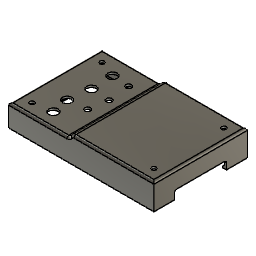
top command (Autodesk Fusion 360 design; units mm, degrees)
Autodesk Fusion 360 part; units mm, degrees
sketch "Esquisse1" plane through (0, 0, 0) normal (0, 0, 1) x (1, 0, 0)
  line L0 (-14.2692, 23.2767) -> (125.7308, 23.2767)
  line L1 (125.7308, 23.2767) -> (125.7308, -66.7233)
  line L2 (125.7308, -66.7233) -> (-14.2692, -66.7233)
  line L3 (-14.2692, -66.7233) -> (-14.2692, 23.2767)
  dimension "d1" = 140
  dimension "d2" = 90
  constraint horizontal L0
  constraint vertical L1
  constraint horizontal L2
  constraint vertical L3
  measures "d1" distance of L0.start L0.end
  measures "d2" distance of L0 L2
extrude "Extrusion1" add sketch "Esquisse1" along normal blind 21
sketch "Esquisse2" plane through (0, 0, 21) normal (0, 0, 1) x (-1, 0, 0)
  line L0 (14.2692, 66.7233) -> (-125.7308, 66.7233)
  line L1 (-125.7308, 66.7233) -> (-125.7308, -23.2767)
  line L2 (-125.7308, -23.2767) -> (14.2692, -23.2767)
  line L3 (14.2692, -23.2767) -> (14.2692, 66.7233)
  line L4 (-125.7308, -23.2767) -> (-45.7308, -23.2767)
  line L5 (-45.7308, -23.2767) -> (-45.7308, 66.7233)
  line L6 (-45.7308, 66.7233) -> (-125.7308, 66.7233)
  line L7 (-125.7308, 66.7233) -> (-125.7308, -23.2767)
  dimension "d5" = 80
  constraint horizontal L4
  constraint vertical L5
  constraint horizontal L6
  constraint vertical L7
  constraint coincident L1.end L2.start
  measures "d5" distance of L1.end L4.end
extrude "Extrusion2" add sketch "Esquisse2" along normal blind 4 contours L0 L1 L2 L4 L5 L6 L7
sketch "Esquisse3" plane through (0, 0, 0) normal (0, 0, -1) x (1, 0, 0)
  line L0 (125.7308, 66.7233) -> (-14.2692, 66.7233)
  line L1 (-14.2692, 66.7233) -> (-14.2692, -23.2767)
  line L2 (-14.2692, -23.2767) -> (125.7308, -23.2767)
  line L3 (125.7308, -23.2767) -> (125.7308, 66.7233)
  line L4 (-12.2692, -21.2767) -> (123.7308, -21.2767)
  line L5 (123.7308, -21.2767) -> (123.7308, 64.7233)
  line L6 (123.7308, 64.7233) -> (-12.2692, 64.7233)
  line L7 (-12.2692, 64.7233) -> (-12.2692, -21.2767)
  dimension "d8" = -2
extrude "Extrusion3" cut sketch "Esquisse3" against normal blind 19 contours L4 L5 L6 L7
sketch "Esquisse4" plane through (0, 0, 19) normal (0, 0, -1) x (1, 0, 0)
  line L0 (-12.2692, 64.7233) -> (-12.2692, -21.2767)
  line L1 (-12.2692, -21.2767) -> (123.7308, -21.2767)
  line L2 (123.7308, -21.2767) -> (123.7308, 64.7233)
  line L3 (123.7308, 64.7233) -> (-12.2692, 64.7233)
  line L4 (123.7308, 64.7233) -> (47.7308, 64.7233)
  line L5 (47.7308, 64.7233) -> (47.7308, -21.2767)
  line L6 (47.7308, -21.2767) -> (123.7308, -21.2767)
  line L7 (123.7308, -21.2767) -> (123.7308, 64.7233)
  dimension "d11" = 76
  constraint horizontal L4
  constraint vertical L5
  constraint horizontal L6
  constraint vertical L7
  constraint coincident L2.end L3.start
  measures "d11" distance of L2.end L4.end
extrude "Extrusion4" cut sketch "Esquisse4" against normal blind 4 contours L1 L2 L3 L4 L5 L6 L7
sketch "Esquisse5" plane through (0, 21.2767, 0) normal (0, -1, 0) x (1, 0, 0)
  line L0 (-12.2692, 0) -> (123.7308, 0)
  line L1 (123.7308, 0) -> (123.7308, 23)
  line L2 (123.7308, 23) -> (47.7308, 23)
  line L3 (47.7308, 23) -> (47.7308, 19)
  line L4 (47.7308, 19) -> (-12.2692, 19)
  line L5 (-12.2692, 19) -> (-12.2692, 0)
  line L6 (-12.2692, 0) -> (123.7308, 0)
  line L7 (123.7308, 0) -> (123.7308, 1)
  line L8 (123.7308, 1) -> (-12.2692, 1)
  line L9 (-12.2692, 1) -> (-12.2692, 0)
  dimension "d14" = 136
  dimension "d15" = 1
  constraint horizontal L6
  constraint vertical L7
  constraint horizontal L8
  constraint vertical L9
  constraint coincident L0.start L5.end
  measures "d14" distance of L0.start L0.end
  measures "d15" distance of L6 L8
extrude "Extrusion5" add sketch "Esquisse5" along normal blind 2 contours L0 L1 L5 L6 L7 L8 L9
sketch "Esquisse6" plane through (0, 19.2767, 0) normal (0, -1, 0) x (1, 0, 0)
  line L0 (-12.2692, 1) -> (-12.2692, 0)
  line L1 (-12.2692, 0) -> (123.7308, 0)
  line L2 (123.7308, 0) -> (123.7308, 1)
  line L3 (123.7308, 1) -> (-12.2692, 1)
  line L4 (123.7308, 1) -> (121.7308, 1)
  line L5 (121.7308, 1) -> (121.7308, 0)
  line L6 (121.7308, 0) -> (123.7308, 0)
  line L7 (123.7308, 0) -> (123.7308, 1)
  dimension "d18" = 2
  constraint horizontal L4
  constraint vertical L5
  constraint horizontal L6
  constraint vertical L7
  constraint coincident L2.end L3.start
  measures "d18" distance of L2.end L4.end
extrude "Extrusion6" add sketch "Esquisse6" along normal blind 84 contours L1 L2 L3 L4 L5 L6 L7
sketch "Esquisse7" plane through (0, 19.2767, 0) normal (0, -1, 0) x (1, 0, 0)
  line L0 (121.7308, 0) -> (121.7308, 1)
  line L1 (121.7308, 1) -> (-12.2692, 1)
  line L2 (-12.2692, 1) -> (-12.2692, 0)
  line L3 (-12.2692, 0) -> (121.7308, 0)
  line L4 (-12.2692, 1) -> (-10.2692, 1)
  line L5 (-10.2692, 1) -> (-10.2692, 0)
  line L6 (-10.2692, 0) -> (-12.2692, 0)
  line L7 (-12.2692, 0) -> (-12.2692, 1)
  dimension "d21" = 2
  constraint horizontal L4
  constraint vertical L5
  constraint horizontal L6
  constraint vertical L7
  constraint coincident L1.end L2.start
  measures "d21" distance of L1.end L4.end
extrude "Extrusion7" add sketch "Esquisse7" along normal blind 84 contours L1 L2 L3 L4 L5 L6 L7
sketch "Esquisse8" plane through (-10.2692, 0, 0) normal (1, 0, 0) x (0, 1, 0)
  line L0 (19.2767, 0) -> (19.2767, 1)
  line L1 (19.2767, 1) -> (-64.7233, 1)
  line L2 (-64.7233, 1) -> (-64.7233, 0)
  line L3 (-64.7233, 0) -> (19.2767, 0)
  line L4 (-64.7233, 1) -> (-62.7233, 1)
  line L5 (-62.7233, 1) -> (-62.7233, 0)
  line L6 (-62.7233, 0) -> (-64.7233, 0)
  line L7 (-64.7233, 0) -> (-64.7233, 1)
  dimension "d24" = 2
  constraint horizontal L4
  constraint vertical L5
  constraint horizontal L6
  constraint vertical L7
  constraint coincident L1.end L2.start
  measures "d24" distance of L1.end L4.end
extrude "Extrusion8" add sketch "Esquisse8" along normal blind 132 contours L1 L2 L3 L4 L5 L6 L7
chamfer "Chanfrein1" distance 2 angle 45 4 edges at (-12.2692, -21.7233, 1) (55.7308, -64.7233, 1) (55.7308, 21.2767, 1) (123.7308, -21.7233, 1)
fillet "Congé1" radius 4 4 edges at (47.7308, -21.7233, 23) (45.7308, -21.7233, 25) (45.7308, -21.7233, 21) (47.7308, -21.7233, 19)
fillet "Congé2" radius 2 10 edges at (87.1949, 23.2767, 25) (46.659, 23.2767, 24.4641) (43.7308, 23.2767, 21.5359) (13.7308, 23.2767, 21) (125.7308, -21.7233, 25) (13.7308, -66.7233, 21) (43.7308, -66.7233, 21.5359) (46.659, -66.7233, 24.4641) (87.1949, -66.7233, 25) (-14.2692, -21.7233, 21)
sketch "Esquisse9" plane through (125.7308, 0, 0) normal (1, 0, 0) x (0, 1, 0)
  line L0 (23.2767, 23) -> (-66.7233, 23)
  line L1 (-66.7233, 23) -> (-66.7233, 0)
  line L2 (-66.7233, 0) -> (23.2767, 0)
  line L3 (23.2767, 0) -> (23.2767, 23)
  line L4 (-44.7233, 8) -> (1.2767, 8)
  line L5 (3.2767, 6) -> (3.2767, 0)
  line L6 (3.2767, 0) -> (-46.7233, 0)
  line L7 (-46.7233, 0) -> (-46.7233, 6)
  arc A0 (-44.7233, 8) -> (-46.7233, 6) centre (-44.7233, 6) ccw
  arc A1 (3.2767, 6) -> (1.2767, 8) centre (1.2767, 6) ccw
  dimension "d32" = 20
  dimension "d33" = 20
  dimension "d34" = 8
  dimension "d35" = 2
  constraint vertical L5
  constraint horizontal L6
  constraint vertical L7
  constraint coincident L2 L5.end
  constraint tangent L4 A0
  constraint tangent L7 A0
  constraint tangent L4 A1
  constraint tangent L5 A1
  constraint equal A0 A1
  measures "d32" distance of L1 L7
  measures "d33" distance of L3 L5
  measures "d34" distance of L4 L6
  measures "d35" radius of A0
extrude "Extrusion9" cut sketch "Esquisse9" against normal blind 25 contours L2 L4 L5 L6 L7 A0 A1
sketch "Esquisse12" plane through (0, 0, 25) normal (0, 0, 1) x (-1, 0, 0)
  line L0 (-48.659, 64.7233) -> (-123.7308, 64.7233)
  line L1 (-123.7308, 64.7233) -> (-123.7308, -21.2767)
  line L2 (-123.7308, -21.2767) -> (-48.659, -21.2767)
  line L3 (-48.659, -21.2767) -> (-48.659, 64.7233)
  circle A0 centre (-114.4808, 55.4733) radius 2.25
  circle A1 centre (-114.4808, -12.0267) radius 2.25
  dimension "d39" = 4.5
  dimension "d40" = 9.25
  dimension "d41" = 9.25
  dimension "d42" = 4.5
  dimension "d43" = 9.25
  dimension "d44" = 9.25
  measures "d39" diameter of A0
  measures "d40" distance of L0 A0.centre
  measures "d41" distance of L1 A0.centre
  measures "d42" diameter of A1
  measures "d43" distance of L1 A1.centre
  measures "d44" distance of L2 A1.centre
extrude "Extrusion10" cut sketch "Esquisse12" against normal blind 2 contours A0 | A1
sketch "Esquisse13" plane through (0, 0, 21) normal (0, 0, 1) x (-1, 0, 0)
  line L0 (12.2692, 64.7233) -> (-41.7308, 64.7233)
  line L1 (-41.7308, 64.7233) -> (-41.7308, -21.2767)
  line L2 (-41.7308, -21.2767) -> (12.2692, -21.2767)
  line L3 (12.2692, -21.2767) -> (12.2692, 64.7233)
  circle A0 centre (3.0192, -12.0267) radius 2.25
  circle A1 centre (3.0192, 55.4733) radius 2.25
  dimension "d47" = 4.5
  dimension "d48" = 9.25
  dimension "d49" = 9.25
  dimension "d50" = 4.5
  dimension "d51" = 9.25
  dimension "d52" = 9.25
  measures "d47" diameter of A0
  measures "d48" distance of L2 A0.centre
  measures "d49" distance of L3 A0.centre
  measures "d50" diameter of A1
  measures "d51" distance of L0 A1.centre
  measures "d52" distance of L3 A1.centre
extrude "Extrusion11" cut sketch "Esquisse13" against normal blind 2 contours A0 | A1
sketch "Esquisse14" plane through (0, 0, 21) normal (0, 0, 1) x (-1, 0, 0)
  circle A0 centre (3.0192, -12.0267) radius 2.25
  circle A1 centre (3.0192, 55.4733) radius 2.25
  line L0 (12.2692, 64.7233) -> (-41.7308, 64.7233)
  line L1 (-41.7308, 64.7233) -> (-41.7308, -21.2767)
  line L2 (-41.7308, -21.2767) -> (12.2692, -21.2767)
  line L3 (12.2692, -21.2767) -> (12.2692, 64.7233)
  circle A2 centre (-11.4424, 36.0698) radius 4.5
  circle A3 centre (-14.6855, 52.5389) radius 4.5
  circle A4 centre (-13.9885, 15.1689) radius 4.5
  circle A5 centre (-13.1269, -5.8406) radius 4.5
  circle A6 centre (-29.6614, -4.9887) radius 2.75
  circle A7 centre (-31.9357, 16.1471) radius 2.75
  circle A8 centre (-29.1937, 34.1072) radius 2.75
  dimension "d55" = 9
  dimension "d56" = 9
  dimension "d57" = 9
  dimension "d58" = 9
  dimension "d59" = 5.5
  dimension "d60" = 5.5
  dimension "d61" = 5.5
  measures "d55" diameter of A2
  measures "d56" diameter of A3
  measures "d57" diameter of A4
  measures "d58" diameter of A5
  measures "d59" diameter of A6
  measures "d60" diameter of A7
  measures "d61" diameter of A8
extrude "Extrusion12" cut sketch "Esquisse14" against normal blind 2 contours A2 | A3 | A4 | A5 | A6 | A7 | A8
